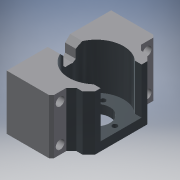
# Autodesk Inventor part: Block Enc
Saved by Autodesk Inventor 2016 (Build 200138000, 138)
## iProperties
Created: 2015-06-11
Part Number: Block Enc
Material: Générique
Document SubType Name: Modeling
Designer: Logan
Density: 1 g/cm^3
Appearance: Par défaut
Author: Logan
Autodesk Inventor part; units mm, degrees
ref_plane "YZ Plane" through (0, 0, 0) normal (1, 0, 0) x (0, 1, 0)
ref_plane "XZ Plane" through (0, 0, 0) normal (0, 1, 0) x (-1, 0, 0)
ref_plane "XY Plane" through (0, 0, 0) normal (0, 0, 1) x (1, 0, 0)
sketch "Esquisse1" plane through (0, 0, 0) normal (0, 0, 1) x (1, 0, 0)
  line L0 (-30, 40) -> (30, 40)
  line L1 (30, 40) -> (30, -40)
  line L2 (30, -40) -> (-30, -40)
  line L3 (-30, -40) -> (-30, 40)
  point P0 (0, 0)
  dimension "d0" = 60
  dimension "d1" = 30
  dimension "d2" = 80
  dimension "d3" = 40
  constraints: 8 end point, 2 parallel, 1 horizontal, 1 perpendicular
  measures "d0" distance between parallel lines of L1 L3
  measures "d1" distance from line of point (0, 0) L3
  measures "d2" distance between parallel lines of L2 L0
  measures "d3" distance from line of point (0, 0) L2
extrude "Extrusion1" add sketch "Esquisse1" along normal blind 40
sketch "Esquisse6" plane through (0, 0, 40) normal (0, 0, 1) x (1, 0, 0)
  arc A0 (24.5516, 16.5) -> (24.5516, -16.5) centre (10, 0) ccw
  line L0 (30, 40) -> (-30, 40) projected
  line L1 (30, -40) -> (30, 40) projected
  line L2 (30, 16.5) -> (24.5516, 16.5)
  line L3 (24.5516, -16.5) -> (30, -16.5)
  line L4 (-30, -40) -> (30, -40) projected
  dimension "d88" = 44
  dimension "d89" = 40
  dimension "d90" = 20
  constraints: 4 end point, 2 horizontal, 2 point on circle, 2 point on line, 1 centre point
  measures "d88" diameter of A0
  measures "d89" distance from line of L0 A0.centre
  measures "d90" distance from line of A0.centre L1
extrude "Extrusion6" cut sketch "Esquisse6" against normal blind 34
sketch "Esquisse12" plane through (0, 0, 6) normal (0, 0, 1) x (1, 0, 0)
  circle A0 centre (10, 0) radius 11
  arc A1 (24.5516, 16.5) -> (24.5516, -16.5) centre (10, 0) ccw projected
  point P0 (0, 0)
  dimension "d93" = 22
  constraints: 1 centre point, 1 concentric
  measures "d93" diameter of A0
extrude "Extrusion11" cut sketch "Esquisse12" against normal up to surface (6 mm away)
sketch "Esquisse13" plane through (0, 0, 0) normal (0, 0, -1) x (-1, 0, 0)
  circle A0 centre (-10, 0) radius 11 projected
  line L0 (30, 40) -> (-30, 40) projected
  line L1 (-30, 40) -> (-30, -40) projected
  line L2 (-30, -40) -> (30, -40) projected
  line L3 (30, -40) -> (30, 40) projected
  arc A1 (-25, 0) -> (-2.5, -12.9904) centre (-10, 0) ccw
  line L4 (-10, 0) -> (-2.5, -12.9904) construction
  line L5 (-10, 0) -> (-25, 0) construction
  arc A2 (-2.5, 12.9904) -> (-25, 0) centre (-10, 0) ccw
  line L6 (-10, 0) -> (-2.5, 12.9904) construction
  line L7 (-10, 0) -> (-25, 0) construction
  point P0 (0, 0)
  dimension "d96" = 15
  dimension "d97" = 120
  dimension "d98" = 15
  dimension "d99" = 120
  constraints: 8 end point, 4 point on circle, 2 centre point, 2 coincident
  measures "d96" radius of A1
  measures "d97" angle of L5 L4
  measures "d98" radius of A2
  measures "d99" angle of L6 L7
hole "Perçage2" at (2.5, 12.9904, 0) at (25, 0, 0) at (2.5, -12.9904, 0) direction (0, 0, 1) diameter 4 end through all counterbore diameter 6 counterbore depth 2
sketch "Esquisse14" plane through (30, -40, 0) normal (1, 0, 0) x (0, 0, -1)
  line L0 (-40, 0) -> (-40, 23.5) projected
  line L1 (0, 0) -> (-40, 0)
  line L2 (-40, 0) -> (-40, 14)
  line L3 (-40, 14) -> (0, 14)
  line L4 (0, 14) -> (0, 0)
  line L5 (-40, 56.5) -> (-40, 80) projected
  line L6 (0, 80) -> (-40, 80)
  line L7 (-40, 80) -> (-40, 66)
  line L8 (-40, 66) -> (0, 66)
  line L9 (0, 66) -> (0, 80)
  point P0 (0, 40)
  dimension "d107" = 14
  dimension "d108" = 14
  constraints: 16 end point, 4 parallel, 2 horizontal, 2 perpendicular, 2 point on line
  measures "d107" distance between parallel lines of L1 L3
  measures "d108" distance between parallel lines of L6 L8
extrude "Extrusion12" cut sketch "Esquisse14" against normal blind 14
chamfer "Chanfrein5" distance 5 angle 45 2 edges at (30, -26, 20) (30, 26, 20)
chamfer "Chanfrein6" distance 4 angle 45 2 edges at (16, -26, 20) (16, 26, 20)
sketch "Esquisse15" plane through (-30, -40, 0) normal (-1, 0, 0) x (0, 0, 1)
  line L0 (0, 0) -> (0, 80) projected
  line L1 (0, 0) -> (40, 0) projected
  line L2 (40, 80) -> (40, 0) projected
  line L3 (0, 80) -> (40, 80) projected
  line L4 (6, 5) -> (35, 5)
  line L5 (35, 75) -> (6, 75)
  line L6 (35, 75) -> (6, 75)
  line L7 (6, 75) -> (6, 5)
  line L8 (6, 5) -> (35, 5)
  line L9 (18, 75) -> (36, 75)
  line L10 (36, 75) -> (36, 5)
  line L11 (36, 5) -> (18, 5)
  point P0 (0, 40)
  point P1 (5, 75)
  point P2 (5, 5)
  constraints: 16 end point, 2 horizontal, 2 parallel, 2 perpendicular, 1 point on line
move faces "Déplacer4" translate (12, 0, 0) faces at (-30, -13.3333, 13.3333)
move faces "Déplacer5" translate (-2, 0, 0) faces at (-18, -13.3333, 13.3333)
sketch "Esquisse16" plane through (-20, -40, 0) normal (-1, 0, 0) x (0, 0, 1)
  line L0 (40, 45) -> (30, 45)
  line L1 (30, 45) -> (30, 35)
  line L2 (30, 35) -> (40, 35)
  line L3 (40, 35) -> (40, 45)
  line L4 (40, 80) -> (40, 0) projected
  point P0 (0, 40)
  dimension "d131" = 10
  dimension "d132" = 10
  dimension "d133" = 5
  constraints: 8 end point, 2 parallel, 1 collinear, 1 horizontal, 1 perpendicular
  measures "d131" distance of L0.end L1.end
  measures "d132" distance of L0.start L0.end
  measures "d133" distance from line of point (0, 40) L0
extrude "Extrusion13" cut sketch "Esquisse16" against normal blind 10
chamfer "Chanfrein7" distance 2 angle 45 2 edges at (-15.7121, 5, 30) (-15.7121, -5, 30)
sketch "Esquisse17" plane through (0, 0, 40) normal (0, 0, 1) x (1, 0, 0)
  line L0 (-20, 5) -> (-11.4243, 5) projected
  arc A0 (24.5516, 16.5) -> (-11.4243, 5) centre (10, 0) ccw projected
  line L1 (24.5516, 16.5) -> (30, 16.5) projected
  line L2 (30, 16.5) -> (30, 21) projected
  line L3 (25, 26) -> (30, 21) projected
  line L4 (25, 26) -> (20, 26) projected
  line L5 (16, 30) -> (20, 26) projected
  line L6 (16, 30) -> (16, 40) projected
  line L7 (16, 40) -> (-20, 40) projected
  line L8 (-20, 40) -> (-20, 5) projected
  line L9 (-11.4243, -5) -> (-20, -5) projected
  line L10 (-20, -5) -> (-20, -40) projected
  line L11 (-20, -40) -> (16, -40) projected
  line L12 (16, -40) -> (16, -30) projected
  line L13 (20, -26) -> (16, -30) projected
  line L14 (20, -26) -> (25, -26) projected
  line L15 (30, -21) -> (25, -26) projected
  line L16 (30, -21) -> (30, -16.5) projected
  line L17 (30, -16.5) -> (24.5516, -16.5) projected
  arc A1 (-11.4243, -5) -> (24.5516, -16.5) centre (10, 0) ccw projected
  point P0 (0, 0)
extrude "Extrusion14" add sketch "Esquisse17" along normal blind 2
sketch "Esquisse18" plane through (-20, -40, 0) normal (0, -1, 0) x (1, 0, 0)
  line L0 (36, 0) -> (36, 42) projected
  line L1 (0, 42) -> (36, 42) projected
  line L2 (0, 0) -> (0, 42) projected
  line L3 (36, 0) -> (0, 0) projected
  point P0 (20, 0)
extrude "Extrusion15" add sketch "Esquisse18" along normal blind 2
sketch "Esquisse19" plane through (-20, 40, 0) normal (0, 1, 0) x (1, 0, 0)
  line L0 (36, -42) -> (36, 0) projected
  line L1 (0, 0) -> (36, 0) projected
  line L2 (0, 0) -> (0, -42) projected
  line L3 (36, -42) -> (0, -42) projected
  point P0 (20, 0)
extrude "Extrusion16" add sketch "Esquisse19" along normal blind 2
sketch "Esquisse20" plane through (0, 0, 0) normal (0, 0, -1) x (-1, 0, 0)
  line L0 (-30, 21) -> (-25, 26) projected
  line L1 (-30, 21) -> (-30, -21) projected
  line L2 (-25, -26) -> (-30, -21) projected
  line L3 (-25, -26) -> (-20, -26) projected
  line L4 (-16, -30) -> (-20, -26) projected
  line L5 (-16, -30) -> (-16, -42) projected
  line L6 (20, -42) -> (-16, -42) projected
  line L7 (20, -42) -> (20, 42) projected
  line L8 (-16, 42) -> (20, 42) projected
  line L9 (-16, 30) -> (-16, 42) projected
  line L10 (-20, 26) -> (-16, 30) projected
  line L11 (-20, 26) -> (-25, 26) projected
  circle A0 centre (-25, 0) radius 3 projected
  circle A1 centre (-2.5, 12.9904) radius 3 projected
  circle A2 centre (-2.5, -12.9904) radius 3 projected
  circle A3 centre (-10, 0) radius 11 projected
  point P0 (0, 0)
extrude "Extrusion17" add sketch "Esquisse20" along normal blind 1
sketch "Esquisse21" plane through (0, 0, 42) normal (0, 0, 1) x (1, 0, 0)
  line L0 (-11.4243, -5) -> (-20, -5) projected
  line L1 (-20, -5) -> (-20, -42) projected
  line L2 (16, -42) -> (-20, -42) projected
  line L3 (16, -30) -> (16, -42) projected
  line L4 (16, -30) -> (20, -26) projected
  line L5 (20, -26) -> (25, -26) projected
  line L6 (25, -26) -> (30, -21) projected
  line L7 (30, -21) -> (30, -16.5) projected
  line L8 (30, -16.5) -> (24.5516, -16.5) projected
  arc A0 (-11.4243, -5) -> (24.5516, -16.5) centre (10, 0) ccw projected
  line L9 (-20, 5) -> (-11.4243, 5) projected
  arc A1 (24.5516, 16.5) -> (-11.4243, 5) centre (10, 0) ccw projected
  line L10 (24.5516, 16.5) -> (30, 16.5) projected
  line L11 (30, 16.5) -> (30, 21) projected
  line L12 (30, 21) -> (25, 26) projected
  line L13 (25, 26) -> (20, 26) projected
  line L14 (20, 26) -> (16, 30) projected
  line L15 (16, 30) -> (16, 42) projected
  line L16 (-20, 42) -> (16, 42) projected
  line L17 (-20, 5) -> (-20, 42) projected
  point P0 (0, 0)
extrude "Extrusion18" add sketch "Esquisse21" along normal blind 1
hole "Perçage4" at (-30, -35, 6) at (-30, 35, 6) at (-30, 35, 36) at (-30, -35, 36) direction (1, 0, 0) diameter 7 depth 60 tip angle 118
chamfer "Chanfrein9" distance 4 angle 45 1 edges at (-15.7121, -5, 43)
chamfer "Chanfrein10" distance 4 angle 45 1 edges at (-15.7121, 5, 43)
chamfer "Chanfrein11" distance 2 angle 45 1 edges at (16, 42, 21)
chamfer "Chanfrein12" distance 2 angle 45 1 edges at (16, -42, 21)
